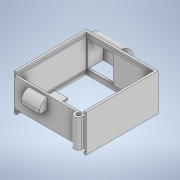
# Autodesk Inventor part: PMS3003
Saved by Autodesk Inventor 2020.3 (Build 243373000, 373)
## iProperties
Created: 2021-02-11
Part Number: PMS3003
Material: Ogólny
Document SubType Name: Modeling
Designer: sitar
Density: 1 g/cm^3
Appearance: Domyślna
Author: sitar
Autodesk Inventor part; units mm, degrees
ref_plane "YZ Plane" through (0, 0, 0) normal (1, 0, 0) x (0, 1, 0)
ref_plane "XY Plane" through (0, 0, 0) normal (0, 0, 1) x (1, 0, 0)
sketch "Szkic1" plane through (0, 0, 0) normal (0, 1, 0) x (-1, 0, 0)
  line L0 (27.5, -27.5) -> (-27.5, -27.5)
  line L1 (-27.5, -27.5) -> (-27.5, 27.5)
  line L2 (-27.5, 27.5) -> (27.5, 27.5)
  line L3 (27.5, 27.5) -> (27.5, -27.5)
  line L4 (27.5, -27.5) -> (-27.5, 27.5) construction
  line L5 (-27.5, -27.5) -> (27.5, 27.5) construction
  point P0 (0, 0)
  dimension "d0" = 55
  dimension "d1" = 55
  constraints: 12 end point, 2 midpoint, 2 parallel, 1 horizontal, 1 perpendicular
  measures "d0" distance of L1.end L2.end
  measures "d1" distance of L0.end L1.end
extrude "Wyciągnięcie proste1" add sketch "Szkic1" along normal blind 23.2
sketch "Szkic8" plane through (-27.5, 0, 27.5) normal (0, 0, 1) x (1, 0, 0)
  line L0 (55, 23.2) -> (53.4, 23.2)
  line L1 (55, 23.2) -> (0, 23.2) projected
  line L2 (55, 0) -> (0, 0) projected
  line L3 (53.4, 23.2) -> (47, 23.2)
  line L4 (47, 23.2) -> (47, 0)
  line L5 (47, 0) -> (53.4, 0)
  line L6 (53.4, 0) -> (53.4, 23.2)
  point P0 (27.5, 0)
  dimension "d50" = 1.6
  dimension "d51" = 6.4
  constraints: 10 end point, 2 parallel, 2 point on line, 1 horizontal, 1 perpendicular
  measures "d50" distance of L0.start L0.end
  measures "d51" distance of L5.end L4.end
extrude "Wyciągnięcie proste6" cut sketch "Szkic8" along normal blind 10
shell "Skorupa2" thickness 1.6 removed faces 1 at (9.1667, 23.2, 9.1667)
sketch "Szkic12" plane through (-27.5, 0, 27.5) normal (0, 0, 1) x (1, 0, 0)
  line L0 (55, 0) -> (55, 23.2) projected
  line L1 (55, 23.2) -> (53.4, 23.2)
  line L2 (55, 23.2) -> (0, 23.2) projected
  line L3 (55, 23.2) -> (56.6, 23.2) construction
  line L4 (1.6, 23.2) -> (53.4, 23.2) projected
  line L5 (55, 0) -> (0, 0) projected
  line L6 (53.4, 23.2) -> (47, 23.2)
  line L7 (47, 23.2) -> (47, 0)
  line L8 (47, 0) -> (53.4, 0)
  line L9 (53.4, 0) -> (53.4, 23.2)
  point P0 (27.5, 0)
  dimension "d73" = 1.6
  dimension "d74" = 180
  dimension "d75" = 6.4
  constraints: 12 end point, 2 collinear, 2 horizontal, 2 parallel, 1 perpendicular, 1 point on line
  measures "d73" distance of L0.end L1.end
  measures "d74" angle of L1 L3
  measures "d75" distance of L8.end L7.end
extrude "Wyciągnięcie proste10" add sketch "Szkic12" along normal blind 1.6 contours L5 L7 L2 L9
sketch "Szkic13" plane through (0, 23.2, 0) normal (0, 1, 0) x (1, 0, 0)
  line L0 (19.5, -28.3) -> (19.5, -29.1) projected
  line L1 (19.5, -29.1) -> (25.9, -29.1) projected
  line L2 (19.5, -29.1) -> (25.9, -29.1)
  line L3 (19.5, -29.1) -> (19.5, -32.3) projected
  line L4 (25.9, -27.5) -> (25.9, -29.1) projected
  arc A0 (19.5, -29.1) -> (25.9, -29.1) centre (22.7, -28.3751) ccw
  point P0 (0, 0)
  dimension "d78" = 3.2811
  constraints: 2 end point, 2 point on circle, 1 centre point, 1 collinear
  measures "d78" radius of A0
extrude "Wyciągnięcie proste11" add sketch "Szkic13" against normal up to surface (23.2 mm away)
sketch "Szkic14" plane through (0, 23.2, 0) normal (0, 1, 0) x (1, 0, 0)
  arc A0 (19.5, -29.1) -> (25.9, -29.1) centre (22.7, -28.3751) ccw projected
  circle A1 centre (22.7, -28.3751) radius 1.6
  point P0 (0, 0)
  dimension "d81" = 3.2
  constraints: 1 centre point, 1 coincident
  measures "d81" diameter of A1
extrude "Wyciągnięcie proste12" cut sketch "Szkic14" against normal through all
sketch "Szkic15" plane through (0, 0, 0) normal (0, -1, 0) x (1, 0, 0)
  line L0 (25.9, 27.5) -> (27.5, 27.5) projected
  line L1 (19.5, 29.1) -> (19.5, 32.3) projected
  line L2 (27.5, 27.5) -> (19.5, 27.5)
  line L3 (19.5, 27.5) -> (19.5, 32.3)
  line L4 (19.5, 32.3) -> (27.5, 32.3)
  line L5 (27.5, 32.3) -> (27.5, 27.5)
  point P0 (0, 0)
  constraints: 8 end point, 2 parallel, 1 horizontal, 1 perpendicular
extrude "Wyciągnięcie proste13" cut sketch "Szkic15" against normal blind 1.6
sketch "Szkic17" plane through (0, 23.2, 0) normal (0, 1, 0) x (1, 0, 0)
  line L0 (-27.5, -27.5) -> (27.5, -27.5) projected
  line L1 (27.5, 27.5) -> (-27.5, 27.5) projected
  line L2 (-27.5, -27.5) -> (-26.7, -27.5)
  line L3 (-26.7, -27.5) -> (-26.7, 27.5)
  line L4 (-26.7, 27.5) -> (-27.5, 27.5)
  line L5 (-27.5, 27.5) -> (-27.5, -27.5)
  line L6 (-27.5, 27.5) -> (27.5, 27.5)
  line L7 (27.5, 27.5) -> (27.5, 26.7)
  line L8 (27.5, 26.7) -> (-27.5, 26.7)
  line L9 (-27.5, 26.7) -> (-27.5, 27.5)
  line L10 (27.5, -27.5) -> (27.5, 27.5) projected
  line L11 (27.5, 27.5) -> (26.7, 27.5)
  line L12 (26.7, 27.5) -> (26.7, -27.5)
  line L13 (26.7, -27.5) -> (27.5, -27.5)
  line L14 (27.5, -27.5) -> (27.5, 27.5)
  point P0 (0, 0)
  point P1 (-26.7, 26.7)
  point P2 (26.7, 26.7)
  dimension "d89" = 0.8
  dimension "d90" = 55
  dimension "d91" = 0.8
  dimension "d92" = 0.8
  dimension "d93" = 55
  constraints: 24 end point, 6 parallel, 3 horizontal, 3 perpendicular, 1 point on line
  measures "d89" distance of L4.end L3.end
  measures "d90" distance of L7.end L8.end
  measures "d91" distance of L6.end L7.end
  measures "d92" distance of L13.end L12.end
  measures "d93" distance of L12.end L11.end
extrude "Wyciągnięcie proste15" add sketch "Szkic17" along normal blind 2 contours L5 L8 L3 L0 | L5 L1 L3 L8 | L12 L8 L10 L0 | L3 L1 L12 L8 | L12 L1 L7 L8
sketch "Szkic18" plane through (0, 25.2, 0) normal (0, 1, 0) x (1, 0, 0)
  line L0 (-27.5, 27.5) -> (-25.9, 27.5)
  line L1 (-25.9, 27.5) -> (-25.9, -27.5)
  line L2 (-25.9, -27.5) -> (-27.5, -27.5)
  line L3 (-27.5, -27.5) -> (-27.5, 27.5)
  line L4 (-27.5, 27.5) -> (27.5, 27.5)
  line L5 (27.5, 27.5) -> (27.5, 25.9)
  line L6 (27.5, 25.9) -> (-27.5, 25.9)
  line L7 (-27.5, 25.9) -> (-27.5, 27.5)
  line L8 (27.5, -27.5) -> (27.5, 27.5) projected
  line L9 (27.5, -27.5) -> (25.9, -27.5)
  line L10 (25.9, -27.5) -> (25.9, 27.5)
  line L11 (25.9, 27.5) -> (27.5, 27.5)
  line L12 (27.5, 27.5) -> (27.5, -27.5)
  point P0 (0, 0)
  point P1 (-25.9, 25.9)
  point P2 (25.9, 25.9)
  dimension "d96" = 1.6
  dimension "d97" = 55
  dimension "d98" = 1.6
  dimension "d99" = 1.6
  dimension "d100" = 55
  constraints: 24 end point, 6 parallel, 3 horizontal, 3 perpendicular
  measures "d96" distance of L1.end L2.end
  measures "d97" distance of L0.end L1.end
  measures "d98" distance of L4.end L5.end
  measures "d99" distance of L10.end L11.end
  measures "d100" distance of L9.end L10.end
extrude "Wyciągnięcie proste16" add sketch "Szkic18" along normal blind 1.2
sketch "Szkic21" plane through (-25.9, 1.6, 25.9) normal (0, 1, 0) x (1, 0, 0)
  line L0 (0, 51.8) -> (0, 0) projected
  line L1 (0, 25.9) -> (0.5, 25.9)
  line L2 (0.5, 25.9) -> (0.5, 30.9)
  line L3 (0.5, 30.9) -> (0, 30.9)
  line L4 (0, 30.9) -> (0, 25.9)
  line L5 (0, 25.9) -> (0.5, 25.9)
  line L6 (0.5, 25.9) -> (0.5, 20.9)
  line L7 (0.5, 20.9) -> (0, 20.9)
  line L8 (0, 20.9) -> (0, 25.9)
  point P0 (25.9, 25.9)
  point P1 (0.5, 25.9)
  dimension "d116" = 0.5
  dimension "d117" = 5
  dimension "d118" = 5
  constraints: 16 end point, 4 parallel, 2 horizontal, 2 perpendicular, 1 midpoint, 1 point on line
  measures "d116" distance of L3.end L2.end
  measures "d117" distance of L2.end L1.end
  measures "d118" distance of L5.end L6.end
extrude "Wyciągnięcie proste19" add sketch "Szkic21" along normal blind 1.2
mirror "Odbij4" about plane through (0, 0, 0) normal (1, 0, 0) of "Wyciągnięcie proste19"
sketch "Szkic22" plane through (-25.9, 1.6, -25.9) normal (0, 1, 0) x (1, 0, 0)
  line L0 (0, 0) -> (4, 0)
  line L1 (4, 0) -> (4, -4)
  line L2 (4, -4) -> (0, -4)
  line L3 (0, -4) -> (0, 0)
  point P0 (25.9, -25.9)
  dimension "d121" = 4
  dimension "d122" = 4
  constraints: 8 end point, 2 parallel, 1 horizontal, 1 perpendicular
  measures "d121" distance of L1.end L2.end
  measures "d122" distance of L0.end L1.end
extrude "Wyciągnięcie proste20" cut sketch "Szkic22" against normal through all
mirror "Odbij5" about plane through (0, 0, 0) normal (1, 0, 0) of "Wyciągnięcie proste20"
mirror "Odbij6" about plane through (0, 0, 0) normal (0, 0, 1) of "Wyciągnięcie proste20", "Odbij5"
sketch "Szkic23" plane through (0, 0, 0) normal (0, -1, 0) x (1, 0, 0)
  line L0 (-27.5, 27.5) -> (27.5, 27.5) projected
  line L1 (27.5, 27.5) -> (27.5, -27.5) projected
  line L2 (-27.5, 27.5) -> (27.5, 27.5)
  line L3 (27.5, 27.5) -> (27.5, -27.5)
  line L4 (27.5, -27.5) -> (-27.5, -27.5)
  line L5 (-27.5, -27.5) -> (-27.5, 27.5)
  point P0 (0, 0)
  constraints: 8 end point, 2 parallel, 1 horizontal, 1 perpendicular
extrude "Wyciągnięcie proste21" cut sketch "Szkic23" against normal blind 1.6
sketch "Szkic24" plane through (0, 1.6, 0) normal (0, -1, 0) x (1, 0, 0)
  line L0 (27.5, 27.5) -> (27.5, -27.5) projected
  line L1 (27.5, -27.5) -> (-27.5, -27.5) projected
  line L2 (27.5, 27.5) -> (26.7, 27.5)
  line L3 (26.7, 27.5) -> (26.7, -27.5)
  line L4 (26.7, -27.5) -> (27.5, -27.5)
  line L5 (27.5, -27.5) -> (27.5, 27.5)
  line L6 (27.5, -27.5) -> (-27.5, -27.5)
  line L7 (-27.5, -27.5) -> (-27.5, -26.7)
  line L8 (-27.5, -26.7) -> (27.5, -26.7)
  line L9 (27.5, -26.7) -> (27.5, -27.5)
  line L10 (-26.7, 27.5) -> (-26.7, -26.7) projected
  line L11 (-27.5, -27.5) -> (-26.7, -27.5)
  line L12 (-26.7, -27.5) -> (-26.7, 27.5)
  line L13 (-26.7, 27.5) -> (-27.5, 27.5)
  line L14 (-27.5, 27.5) -> (-27.5, -27.5)
  point P0 (0, 0)
  point P1 (26.7, -26.7)
  dimension "d127" = 0.8
  dimension "d128" = 55
  dimension "d129" = 55
  constraints: 24 end point, 6 parallel, 3 horizontal, 3 perpendicular, 1 point on line
  measures "d127" distance of L4.end L3.end
  measures "d128" distance of L7.end L8.end
  measures "d129" distance of L10.start L11.end
extrude "Wyciągnięcie proste22" add sketch "Szkic24" along normal blind 2
sketch "Szkic25" plane through (0, -0.4, 0) normal (0, -1, 0) x (1, 0, 0)
  line L0 (27.5, 27.5) -> (27.5, -27.5) projected
  line L1 (27.5, 27.5) -> (25.9, 27.5)
  line L2 (25.9, 27.5) -> (25.9, -27.5)
  line L3 (25.9, -27.5) -> (27.5, -27.5)
  line L4 (27.5, -27.5) -> (27.5, 27.5)
  line L5 (27.5, -27.5) -> (-27.5, -27.5) projected
  line L6 (27.5, -27.5) -> (-27.5, -27.5)
  line L7 (-27.5, -27.5) -> (-27.5, -25.9)
  line L8 (-27.5, -25.9) -> (27.5, -25.9)
  line L9 (27.5, -25.9) -> (27.5, -27.5)
  line L10 (-27.5, -27.5) -> (-27.5, 27.5) projected
  line L11 (-27.5, -27.5) -> (-25.9, -27.5)
  line L12 (-25.9, -27.5) -> (-25.9, 27.5)
  line L13 (-25.9, 27.5) -> (-27.5, 27.5)
  line L14 (-27.5, 27.5) -> (-27.5, -27.5)
  point P0 (0, 0)
  point P1 (25.9, -25.9)
  point P2 (-25.9, -25.9)
  dimension "d132" = 1.6
  dimension "d133" = 55
  dimension "d134" = 55
  dimension "d135" = 1.6
  dimension "d136" = 1.6
  dimension "d137" = 55
  constraints: 24 end point, 6 parallel, 3 horizontal, 3 perpendicular
  measures "d132" distance of L3.end L2.end
  measures "d133" distance of L2.end L1.end
  measures "d134" distance of L7.end L8.end
  measures "d135" distance of L6.end L7.end
  measures "d136" distance of L13.end L12.end
  measures "d137" distance of L12.end L11.end
extrude "Wyciągnięcie proste23" add sketch "Szkic25" along normal blind 1.6
ref_plane "Płaszczyzna konstrukcyjna1" through (0, 22, 0) normal (0, 1, 0) x (-1, 0, 0)
sketch "Szkic26" plane through (0, 1.6, 0) normal (0, -1, 0) x (1, 0, 0)
  line L0 (-25.4, 5) -> (-25.9, 5) projected
  line L1 (-25.9, -5) -> (-25.4, -5) projected
  line L2 (-25.4, 5) -> (-25.9, 5)
  line L3 (-25.9, 5) -> (-25.9, -5)
  line L4 (-25.9, -5) -> (-25.4, -5)
  line L5 (-25.4, -5) -> (-25.4, 5)
  line L6 (25.9, 5) -> (25.4, 5) projected
  line L7 (25.4, -5) -> (25.9, -5) projected
  line L8 (25.4, 5) -> (25.9, 5)
  line L9 (25.9, 5) -> (25.9, -5)
  line L10 (25.9, -5) -> (25.4, -5)
  line L11 (25.4, -5) -> (25.4, 5)
  point P0 (0, 0)
  constraints: 16 end point, 4 parallel, 2 horizontal, 2 perpendicular
extrude "Wyciągnięcie proste24" cut sketch "Szkic26" against normal blind 3
sketch "Szkic29" plane through (19.5, 1.6, 27.5) normal (0, 0, 1) x (1, 0, 0)
  line L0 (-28.4, 16.2) -> (-28.4, 0)
  line L1 (-46.2, 0) -> (0, 0) projected
  line L2 (-28.4, 16.2) -> (-12.2, 16.2) construction
  line L3 (-28.4, 16.2) -> (-45.4, 16.2)
  line L4 (-28.4, 16.2) -> (-11.4, 16.2) construction
  line L5 (-45.4, 0) -> (-45.4, 21.6) projected
  line L6 (-32.9, 18.2) -> (-23.9, 18.2)
  line L7 (-23.9, 18.2) -> (-23.9, 14.2)
  line L8 (-23.9, 14.2) -> (-32.9, 14.2)
  line L9 (-32.9, 14.2) -> (-32.9, 18.2)
  line L10 (-32.9, 18.2) -> (-23.9, 14.2) construction
  line L11 (-23.9, 18.2) -> (-32.9, 14.2) construction
  point P0 (-19.5, -1.6)
  dimension "d155" = 16.2
  dimension "d156" = 90
  dimension "d157" = 17
  dimension "d158" = 180
  dimension "d159" = 9
  dimension "d160" = 4
  constraints: 20 end point, 4 horizontal, 2 equal length, 2 midpoint, 2 parallel, 2 perpendicular, 2 point on line
  measures "d155" distance of L0.start L0.end
  measures "d156" angle of L0 L2
  measures "d157" distance of L0.start L3.end
  measures "d158" angle of L3 L4
  measures "d159" distance of L7.end L8.end
  measures "d160" distance of L6.end L7.end
sketch "Szkic30" plane through (19.5, 1.6, 27.5) normal (0, 0, 1) x (1, 0, 0)
  line L0 (-35.4, 20) -> (-21.4, 20)
  line L1 (-21.4, 20) -> (-21.4, 12)
  line L2 (-21.4, 12) -> (-35.4, 12)
  line L3 (-35.4, 12) -> (-35.4, 20)
  line L4 (-35.4, 20) -> (-45.4, 20)
  line L5 (-35.4, 20) -> (-25.4, 20) construction
  line L6 (-45.4, 0) -> (-45.4, 21.6) projected
  line L7 (-35.4, 20) -> (-35.4, 0)
  line L8 (-35.4, 20) -> (-15.4, 20) construction
  line L9 (-46.2, 0) -> (0, 0) projected
  point P0 (-19.5, -1.6)
  dimension "d161" = 14
  dimension "d162" = 8
  dimension "d163" = 10
  dimension "d164" = 180
  dimension "d165" = 20
  dimension "d166" = 90
  constraints: 16 end point, 4 horizontal, 2 equal length, 2 parallel, 2 point on line, 1 collinear, 1 perpendicular
  measures "d161" distance of L1.end L2.end
  measures "d162" distance of L0.end L1.end
  measures "d163" distance of L0.start L4.end
  measures "d164" angle of L4 L5
  measures "d165" distance of L0.start L7.end
  measures "d166" angle of L7 L8
extrude "Wyciągnięcie proste26" add sketch "Szkic30" along normal blind 6 contours L0 L1 L2 L3
fillet "Zaokrąglenie3" radius 6 1 edges at (-8.9, 21.6, 33.5)
shell "Skorupa4" thickness 1.6 removed faces 1 at (-11.2333, 13.6, 29.5)
extrude "Wyciągnięcie proste27" cut sketch "Szkic29" against normal up to surface (1.6 mm away) contours L3 L9 L6 L7 L8 L0 | L0 L8 L9 L3
sketch "Szkic31" plane through (-4.4, 15.8, 25.9) normal (-1, 0, 0) x (0, 0, 1)
  line L0 (1.6, 4) -> (1.6, 0) projected
  line L1 (0, 4) -> (1.6, 4)
  line L2 (1.6, 4) -> (1.6, 0)
  line L3 (1.6, 0) -> (0, 0)
  line L4 (0, 0) -> (0, 4)
  point P0 (-25.9, -15.8)
  constraints: 8 end point, 2 parallel, 1 horizontal, 1 perpendicular
extrude "Wyciągnięcie proste28" cut sketch "Szkic31" against normal up to surface (0.9 mm away)
sketch "Szkic32" plane through (-13.4, 15.8, 25.9) normal (1, 0, 0) x (0, 0, -1)
  line L0 (-1.6, 4) -> (0, 4) projected
  line L1 (-1.6, 0) -> (-1.6, 4) projected
  line L2 (0, 4) -> (-1.6, 4)
  line L3 (-1.6, 4) -> (-1.6, 0)
  line L4 (-1.6, 0) -> (0, 0)
  line L5 (0, 0) -> (0, 4)
  point P0 (25.9, -15.8)
  constraints: 8 end point, 2 parallel, 1 horizontal, 1 perpendicular
extrude "Wyciągnięcie proste29" cut sketch "Szkic32" against normal up to surface (0.9 mm away)
sketch "Szkic33" plane through (-14.3, 19.8, 25.9) normal (0, -1, 0) x (1, 0, 0)
  line L0 (0, 0) -> (0, 1.6) projected
  line L1 (10.8, 1.6) -> (10.8, 0) projected
  line L2 (0, 0) -> (10.8, 0)
  line L3 (10.8, 0) -> (10.8, 1.6)
  line L4 (10.8, 1.6) -> (0, 1.6)
  line L5 (0, 1.6) -> (0, 0)
  point P0 (14.3, -25.9)
  constraints: 8 end point, 2 parallel, 1 horizontal, 1 perpendicular
extrude "Wyciągnięcie proste30" cut sketch "Szkic33" against normal blind 0.2
sketch "Szkic35" plane through (-25.9, 23.2, -25.9) normal (0, 0, 1) x (1, 0, 0)
  line L0 (1, -1.1) -> (21, -1.1)
  line L1 (21, -1.1) -> (21, -21.1)
  line L2 (21, -21.1) -> (1, -21.1)
  line L3 (1, -21.1) -> (1, -1.1)
  line L4 (1, -21.1) -> (1, -21.6)
  line L5 (51.8, -21.6) -> (0, -21.6) projected
  line L6 (1, -21.1) -> (0, -21.1)
  line L7 (1, -21.1) -> (2, -21.1) construction
  line L8 (0, 0) -> (0, -21.6) projected
  point P0 (25.9, -23.2)
  dimension "d179" = 20
  dimension "d180" = 20
  dimension "d181" = 0.5
  dimension "d182" = 1
  dimension "d183" = 180
  constraints: 14 end point, 3 horizontal, 2 parallel, 2 point on line, 1 collinear, 1 perpendicular, 1 vertical
  measures "d179" distance of L1.end L2.end
  measures "d180" distance of L0.end L1.end
  measures "d181" distance of L2.end L4.end
  measures "d182" distance of L2.end L6.end
  measures "d183" angle of L6 L7
sketch "Szkic37" plane through (27.5, 26.4, -27.5) normal (0, 0, -1) x (-1, 0, 0)
  line L0 (30.8, -2.7) -> (54, -2.7)
  line L1 (54, -2.7) -> (54, -24.3)
  line L2 (54, -24.3) -> (30.8, -24.3)
  line L3 (30.8, -24.3) -> (30.8, -2.7)
  line L4 (54, -24.3) -> (54, -28.4)
  line L5 (55, -28.4) -> (0, -28.4) projected
  line L6 (54, -24.3) -> (58.1, -24.3) construction
  line L7 (54, -24.3) -> (55, -24.3)
  line L8 (55, -28.4) -> (55, 0) projected
  point P0 (27.5, -26.4)
  dimension "d187" = 23.2
  dimension "d188" = 21.6
  dimension "d189" = 4.1
  dimension "d190" = 90
  dimension "d191" = 1
  constraints: 14 end point, 2 horizontal, 2 parallel, 2 perpendicular, 2 point on line, 1 vertical, 2 other
  measures "d187" distance of L1.end L2.end
  measures "d188" distance of L0.end L1.end
  measures "d189" distance of L1.end L4.end
  measures "d190" angle of L4 L6
  measures "d191" distance of L1.end L7.end
extrude "Wyciągnięcie proste31" add sketch "Szkic37" along normal blind 12 contours L0 L1 L2 L3
fillet "Zaokrąglenie4" radius 10 1 edges at (-14.9, 23.7, -39.5)
shell "Skorupa5" thickness 1.6 removed faces 1 at (-11.0333, 2.1, -31.5)
extrude "Wyciągnięcie proste32" cut sketch "Szkic35" against normal up to surface (1.6 mm away) contours L0 L1 L2 L3
sketch "Szkic39" plane through (-26.5, 2.1, -39.5) normal (0, -1, 0) x (1, 0, 0)
  line L0 (1.6, 11.2) -> (21.6, 11.2) projected
  line L1 (21.6, 12) -> (21.6, 11.2) projected
  line L2 (1.6, 11.2) -> (21.6, 11.2)
  line L3 (21.6, 11.2) -> (21.6, 12)
  line L4 (21.6, 12) -> (1.6, 12)
  line L5 (1.6, 12) -> (1.6, 11.2)
  point P0 (26.5, 39.5)
  constraints: 8 end point, 2 parallel, 1 horizontal, 1 perpendicular
extrude "Wyciągnięcie proste33" cut sketch "Szkic39" against normal up to surface (1.1 mm away)
sketch "Szkic43" plane through (0, 22, 0) normal (0, 1, 0) x (-1, 0, 0)
  line L0 (-25.9, 25.9) -> (25.9, 25.9) projected
  line L1 (2, 25.9) -> (-8, 25.9)
  line L2 (-8, 25.9) -> (-8, 21.9)
  line L3 (-8, 21.9) -> (2, 21.9)
  line L4 (2, 21.9) -> (2, 25.9)
  line L5 (2, 25.9) -> (0, 25.9)
  point P0 (0, 0)
  point P1 (-8, 25.9)
  dimension "d211" = 10
  dimension "d212" = 4
  dimension "d213" = 2
  constraints: 10 end point, 2 parallel, 2 point on line, 1 horizontal, 1 midpoint, 1 perpendicular
  measures "d211" distance of L3.end L2.end
  measures "d212" distance of L2.end L1.end
  measures "d213" distance of L5.end L1.start
extrude "Wyciągnięcie proste36" add sketch "Szkic43" along normal blind 1.2
